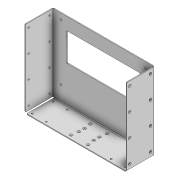
# Autodesk Inventor part: Display_Mount_A
Saved by Autodesk Inventor 2020 (Build 240168000, 168)
## iProperties
Created: 2021-12-05
Part Number: Display_Mount_A
Material: 一般
Document SubType Name: Sheet Metal
Designer: ken113
Density: 1 g/cm^3
Sheet Metal Rule: Default_mm
Appearance: 既定
Author: ken113
Autodesk Inventor part; units mm, degrees
ref_plane "YZ Plane" through (0, 0, 0) normal (1, 0, 0) x (0, 1, 0)
ref_plane "XZ Plane" through (0, 0, 0) normal (0, 1, 0) x (-1, 0, 0)
ref_plane "XY Plane" through (0, 0, 0) normal (0, 0, 1) x (1, 0, 0)
sketch "スケッチ1" plane through (0, 0, 0) normal (0, 0, 1) x (1, 0, 0)
  line L0 (175, -135) -> (-175, -135)
  line L1 (-175, -135) -> (-175, 135)
  line L2 (-175, 135) -> (175, 135)
  line L3 (175, 135) -> (175, -135)
  line L4 (175, -135) -> (-175, 135) construction
  line L5 (-175, -135) -> (175, 135) construction
  point P0 (0, 0)
  dimension "d0" = 270
  dimension "d1" = 350
  measures "d0" distance of L0.end L1.end
  measures "d1" distance of L1.end L2.end
extrude "プレート1" add sketch "スケッチ1" along normal blind 3
sketch "スケッチ2" plane through (175, -138, 6) normal (0, -1, 0) x (1, 0, 0)
  line L0 (-350, 0) -> (0, 0)
  line L1 (0, 0) -> (0, 94)
  line L2 (0, 94) -> (-350, 94)
  line L3 (-350, 94) -> (-350, 0)
  constraints: 6 end point, 1 horizontal, 1 perpendicular, 1 vertical
edge flange "フランジ1" height 100 angle 90 thickness 3 bend radius 3 thickness toward (0, -1, 0) relief straight relief width 3 relief depth 1.5 edges at (0, -135, 3) wall of the first edge with corners at (-175, -138, 6) (175, -138, 6) (175, -138, 100) (-175, -138, 100)
bend "曲げ1"
corner "コーナー1"
sketch "スケッチ3" plane through (0, 0, 3) normal (0, 0, 1) x (1, 0, 0)
  line L0 (150, -85) -> (-150, -85)
  line L1 (-150, -85) -> (-150, 115)
  line L2 (-150, 115) -> (150, 115)
  line L3 (150, 115) -> (150, -85)
  line L4 (150, -85) -> (-150, 115) construction
  line L5 (-150, -85) -> (150, 115) construction
  line L6 (175, -135) -> (-175, -135) projected
  point P0 (0, 0)
  point P1 (0, 15)
  dimension "d13" = 300
  dimension "d14" = 200
  dimension "d15" = 50
  constraints: 12 end point, 2 midpoint, 2 parallel, 1 horizontal, 1 perpendicular
  measures "d13" distance of L0.start L0.end
  measures "d14" distance of L0.end L1.end
  measures "d15" distance between parallel lines of L0 L6
hole "穴1" at (-150, 115, 3) at (-150, -85, 3) at (150, -85, 3) at (150, 115, 3) direction (0, 0, -1) diameter 6.2 depth 3 tip angle 118
sketch "スケッチ4" plane through (0, 0, 3) normal (0, 0, 1) x (1, 0, 0)
  line L0 (130, -8.8) -> (-130, -8.8)
  line L1 (-130, -8.8) -> (-130, 91.2)
  line L2 (-130, 91.2) -> (130, 91.2)
  line L3 (130, 91.2) -> (130, -8.8)
  line L4 (130, -8.8) -> (-130, 91.2) construction
  line L5 (-130, -8.8) -> (130, 91.2) construction
  circle A0 centre (-150, 115) radius 3.1 projected
  point P0 (0, 0)
  point P1 (0, 41.2)
  point P2 (0, 41.2)
  dimension "d23" = 100
  dimension "d24" = 23.8
  dimension "d25" = 260
  constraints: 12 end point, 3 midpoint, 2 parallel, 1 horizontal, 1 perpendicular, 1 vertical alignment
  measures "d23" distance of L2.end L0.start
  measures "d24" distance from line of L2 A0.centre
  measures "d25" distance of L1.end L2.end
extrude "押し出し1" cut sketch "スケッチ4" against normal through all contours L0 L1 L2 L3
fillet "フィレット1" radius 2 4 edges at (130, -8.8, 1.5) (130, 91.2, 1.5) (-130, 91.2, 1.5) (-130, -8.8, 1.5)
sketch "スケッチ5" plane through (-175, -138, 100) normal (0, 1, 0) x (1, 0, 0)
  line L0 (350, 94) -> (0, 94) projected
  line L1 (0, 0) -> (0, 94) projected
  line L2 (0, 0) -> (350, 0) projected
  line L3 (350, 0) -> (350, 94) projected
  line L4 (145, 13) -> (205, 13)
  line L5 (205, 13) -> (205, 81)
  line L6 (205, 81) -> (145, 81)
  line L7 (145, 81) -> (145, 13)
  line L8 (145, 13) -> (205, 81) construction
  line L9 (205, 13) -> (145, 81) construction
  line L10 (148.5, 37) -> (201.5, 37)
  line L11 (201.5, 37) -> (201.5, 57)
  line L12 (201.5, 57) -> (148.5, 57)
  line L13 (148.5, 57) -> (148.5, 37)
  line L14 (148.5, 37) -> (201.5, 57) construction
  line L15 (201.5, 37) -> (148.5, 57) construction
  point P0 (175, 100)
  point P1 (175, 47)
  point P2 (175, 0)
  point P3 (175, 47)
  point P4 (0, 47)
  point P5 (175, 47)
  dimension "d29" = 60
  dimension "d30" = 68
  dimension "d31" = 53
  dimension "d32" = 20
  constraints: 24 end point, 8 midpoint, 4 parallel, 2 horizontal, 2 perpendicular, 1 horizontal alignment, 1 vertical alignment
  measures "d29" distance of L6.end L5.end
  measures "d30" distance of L5.end L4.end
  measures "d31" distance of L12.end L11.end
  measures "d32" distance of L11.end L10.end
hole "穴2" at (-30, -138, 19) at (-26.5, -138, 43) at (-26.5, -138, 63) at (26.5, -138, 63) at (26.5, -138, 43) at (30, -138, 19) at (30, -138, 87) at (-30, -138, 87) direction (0, -1, 0) diameter 5.2 depth 3 tip angle 118 countersink diameter 10 countersink angle 90
sketch "スケッチ6" plane through (178, 135, 6) normal (1, 0, 0) x (0, 1, 0)
  line L0 (-270, 0) -> (0, 0)
  line L1 (0, 0) -> (0, 94)
  line L2 (0, 94) -> (-270, 94)
  line L3 (-270, 94) -> (-270, 0)
  constraints: 6 end point, 1 horizontal, 1 perpendicular, 1 vertical
edge flange "フランジ2" height 100 angle 90 thickness 3 bend radius 3 thickness toward (1, 0, 0) relief straight relief width 3 relief depth 1.5 corner gap 3 corner form 0 edges at (175, 0, 3) (-175, 0, 3) wall of the first edge with corners at (178, -135, 6) (178, 135, 6) (178, 135, 100) (178, -135, 100)
bend "曲げ2"
corner "コーナー2"
fillet "フィレット2" radius 2 6 edges at (-179.5, 135, 100) (-179.5, -135, 100) (-175, -139.5, 100) (175, -139.5, 100) (179.5, -135, 100) (179.5, 135, 100)
sketch "スケッチ7" plane through (181, -135, 6) normal (1, 0, 0) x (0, 0, -1)
  arc A0 (-94, 268) -> (-92, 270) centre (-92, 268) ccw projected
  line L0 (-94, 2) -> (-94, 268) projected
  arc A1 (-92, 0) -> (-94, 2) centre (-92, 2) ccw projected
  line L1 (0, 0) -> (-92, 0) projected
  line L2 (0, 0) -> (0, 270) projected
  line L3 (-92, 270) -> (0, 270)
  line L4 (-10, 255) -> (-10, 15)
  line L5 (-10, 15) -> (-84, 15)
  line L6 (-84, 15) -> (-84, 255)
  line L7 (-84, 255) -> (-10, 255)
  line L8 (-84, 95) -> (-10, 95)
  line L9 (-10, 95) -> (-10, 175)
  line L10 (-10, 175) -> (-84, 175)
  line L11 (-84, 175) -> (-84, 95)
  point P0 (6, 135)
  dimension "d51" = 10
  dimension "d52" = 240
  dimension "d53" = 80
  dimension "d54" = 80
  dimension "d75" = 10
  dimension "d76" = 15
  dimension "d77" = 15
  constraints: 18 end point, 2 centre point, 2 parallel, 2 perpendicular, 2 point on line, 1 horizontal
  measures "d51" distance between parallel lines of L2 L4
  measures "d52" distance of L5.end L6.end
  measures "d53" distance between parallel lines of L7 L10
  measures "d54" distance between parallel lines of L10 L8
  measures "d75" distance between parallel lines of L6 L0
  measures "d76" distance between parallel lines of L5 L1
  measures "d77" distance between parallel lines of L3 L7
hole "穴3" at (181, 120, 90) at (181, 120, 16) at (181, 40, 16) at (181, 40, 90) at (181, -40, 16) at (181, -40, 90) at (181, -120, 90) at (181, -120, 16) direction (-1, 0, 0) diameter 5.2 depth 3 tip angle 118 countersink diameter 10 countersink angle 90
mirror "ミラー1" about plane through (0, 0, 0) normal (1, 0, 0) of "穴3"
sketch "スケッチ8" plane through (-175, -138, 6) normal (0, 1, 0) x (1, 0, 0)
  point P0 (175, 6)
sketch "スケッチ9" plane through (-175, -141, 6) normal (0, -1, 0) x (1, 0, 0)
  arc A0 (350, 92) -> (348, 94) centre (348, 92) ccw projected
  line L0 (2, 94) -> (348, 94) projected
  arc A1 (2, 94) -> (0, 92) centre (2, 92) ccw projected
  line L1 (0, 0) -> (0, 92) projected
  line L2 (0, 0) -> (350, 0) projected
  line L3 (350, 92) -> (350, 0) projected
  circle A2 centre (205, 81) radius 2.6 projected
  circle A3 centre (201.5, 37) radius 2.6 projected
  circle A4 centre (148.5, 57) radius 2.6 projected
  circle A5 centre (145, 13) radius 2.6 projected
  circle A6 centre (148.5, 37) radius 2.6 projected
  circle A7 centre (201.5, 57) radius 2.6 projected
  circle A8 centre (205, 13) radius 2.6 projected
  circle A9 centre (145, 81) radius 2.6 projected
  line L4 (10, 84) -> (60, 84)
  line L5 (60, 84) -> (60, 10)
  line L6 (60, 10) -> (10, 10)
  line L7 (10, 10) -> (10, 84)
  line L8 (290, 84) -> (340, 84)
  line L9 (340, 84) -> (340, 10)
  line L10 (340, 10) -> (290, 10)
  line L11 (290, 10) -> (290, 84)
  point P0 (175, -6)
  dimension "d62" = 10
  dimension "d63" = 10
  dimension "d64" = 10
  dimension "d65" = 10
  dimension "d66" = 50
  dimension "d67" = 50
  constraints: 16 end point, 4 parallel, 2 horizontal, 2 perpendicular, 2 point on line
  measures "d62" distance between parallel lines of L7 L1
  measures "d63" distance between parallel lines of L0 L4
  measures "d64" distance between parallel lines of L6 L2
  measures "d65" distance between parallel lines of L3 L9
  measures "d66" distance of L4.start L4.end
  measures "d67" distance of L8.start L8.end
hole "穴4" at (-165, -141, 16) at (-165, -141, 90) at (-115, -141, 90) at (-115, -141, 16) at (115, -141, 16) at (165, -141, 16) at (165, -141, 90) at (115, -141, 90) direction (0, 1, 0) diameter 5.2 depth 3 tip angle 118 countersink diameter 10 countersink angle 90
equation "\"d21\" = Thickness"
equation "\"d38\" = Thickness"
equation "\"d53\" = 0.333333 * d52"
equation "\"d54\" = d53"
equation "\"d60\" = Thickness"
equation "\"d73\" = Thickness"
equation "\"d2\" = Thickness"
equation "\"d3\" = BendReliefWidth"
equation "\"d4\" = BendReliefDepth"
equation "\"d5\" = MinimumRemnant"
equation "\"d6\" = TransitionRadius"
equation "\"d9\" = BendRadius"
equation "\"d10\" = CornerReliefSize"
equation "\"d11\" = GapSize"
equation "\"d12\" = JacobiRadiusSize"
equation "\"d40\" = BendReliefWidth"
equation "\"d41\" = BendReliefDepth"
equation "\"d42\" = MinimumRemnant"
equation "\"d43\" = TransitionRadius"
equation "\"d46\" = BendRadius"
equation "\"d47\" = CornerReliefSize"
equation "\"d48\" = GapSize"
equation "\"d49\" = JacobiRadiusSize"
equation "\"BendRadius\" = Thickness"
equation "\"BendReliefWidth\" = Thickness"
equation "\"BendReliefDepth\" = 0.5 * Thickness"
equation "\"CornerReliefSize\" = 4 * Thickness"
equation "\"MinimumRemnant\" = 2 * Thickness"
equation "\"TransitionRadius\" = BendRadius"
equation "\"JacobiRadiusSize\" = BendRadius"
equation "\"GapSize\" = Thickness"
equation "\"Thickness\" = 3"
